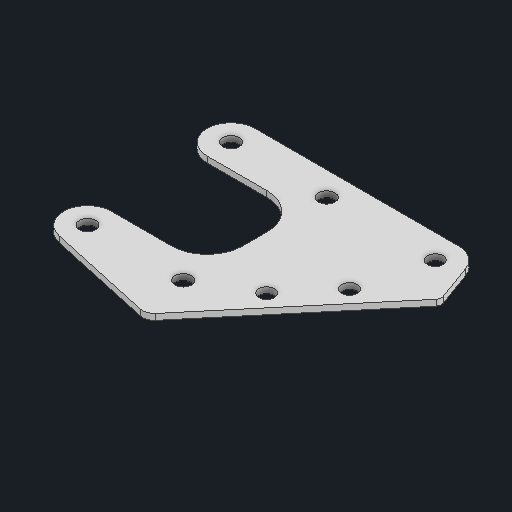
# Autodesk Inventor part: funel_gusset
Saved by Autodesk Inventor 2025 (Build 290162000, 162)
## iProperties
Created: 2024-10-12
Part Number: funel_gusset
Material: Generic
Document SubType Name: Modeling
Designer: Averey Ku
Density: 1 g/cm^3
Appearance: Default
d0: 0.164 in
d1: 0.500 in
d6: 0.375 in
d8: 0.164 in
d9: 0.063 in
d14: 0.164 in
d15: 0.615 in
d17: 0.125 in
Author: Averey Ku
Autodesk Inventor part; units mm, degrees
ref_plane "YZ Plane" through (0, 0, 0) normal (1, 0, 0) x (0, 1, 0)
ref_plane "XZ Plane" through (0, 0, 0) normal (0, 1, 0) x (-1, 0, 0)
ref_plane "XY Plane" through (0, 0, 0) normal (0, 0, 1) x (1, 0, 0)
sketch "main" plane through (0, 0, 0) normal (0, 0, 1) x (1, 0, 0)
  circle A0 centre (-18.9483, -3.9137) radius 2.0828
  arc A1 (-24.9153, -6.0856) -> (-18.95, -10.2637) centre (-18.9483, -3.9137) ccw
  line L0 (5.8565, 45.4052) -> (-28.0879, 4.9518)
  circle A2 centre (9.8531, -3.9215) radius 2.1844
  line L1 (-18.95, -10.2637) -> (35.2514, -10.2783)
  line L2 (9.8472, 18.301) -> (9.8489, 11.9535)
  arc A3 (9.8489, 11.9535) -> (19.3764, 2.4311) centre (19.3739, 11.9561) ccw
  circle A4 centre (9.8531, 34.1785) radius 2.1844
  line L3 (35.2514, 2.4354) -> (19.3764, 2.4311)
  arc A5 (35.2514, -10.2783) -> (35.2514, 2.4354) centre (35.2531, -3.9215) ccw
  circle A6 centre (35.2531, 34.1785) radius 2.1844
  arc A7 (35.2531, 27.8285) -> (36.6181, 40.3801) centre (35.2531, 34.1785) ccw
  circle A8 centre (35.2531, -3.9215) radius 2.1844
  line L4 (-28.3636, 3.3884) -> (-24.9153, -6.0856)
  line L5 (19.3722, 27.8285) -> (35.2531, 27.8285)
  arc A9 (19.3722, 27.8285) -> (9.8472, 18.301) centre (19.3722, 18.3035) ccw
  circle A10 centre (-14.2094, 14.0824) radius 2.0828
  arc A11 (-28.0879, 4.9518) -> (-28.3636, 3.3884) centre (-26.8718, 3.9314) ccw
  circle A12 centre (-4.1684, 26.0488) radius 2.0828
  line L6 (-4.1684, 26.0488) -> (-14.2094, 14.0824)
  line L7 (8.9712, 46.4651) -> (36.6181, 40.3801)
  arc A13 (8.9712, 46.4651) -> (5.8565, 45.4052) centre (8.2887, 43.3643) ccw
  point P0 (9.379, 13.4106)
  point P1 (9.8514, 2.4285)
  point P2 (9.8446, 27.8285)
  dimension "d0" = 4.1656
  dimension "d1" = 12.7
  dimension "d6" = 9.525
  dimension "d8" = 4.1656
  dimension "d9" = 1.5875
  dimension "d14" = 4.1656
  dimension "d15" = 15.621
  dimension "d17" = 3.175
  measures "d0" diameter of A0
  measures "d1" diameter of A1
  measures "d6" radius of A9
  measures "d8" diameter of A10
  measures "d9" radius of A11
  measures "d14" diameter of A12
  measures "d15" distance of L6.start L6.end
  measures "d17" radius of A13
sketch "Sketch1" plane through (0, 0, 0) normal (0, 1, 0) x (-1, 0, 0)
  circle A0 centre (-54.2014, -38.0923) radius 2.0828
  arc A1 (-60.1685, -40.2641) -> (-54.2031, -44.4423) centre (-54.2014, -38.0923) ccw
  line L0 (-29.3966, 11.2266) -> (-63.341, -29.2268)
  circle A2 centre (-25.4, -38.1) radius 2.1844
  line L1 (-54.2031, -44.4423) -> (-0.0017, -44.4568)
  line L2 (-25.406, -15.8776) -> (-25.4043, -22.225)
  arc A3 (-25.4043, -22.225) -> (-15.8767, -31.7474) centre (-15.8793, -22.2224) ccw
  circle A4 centre (-25.4, 0) radius 2.1844
  line L3 (-0.0017, -31.7432) -> (-15.8767, -31.7474)
  arc A5 (-0.0017, -44.4568) -> (-0.0017, -31.7432) centre (0, -38.1) ccw
  circle A6 centre (0, 0) radius 2.1844
  arc A7 (0, -6.35) -> (1.3649, 6.2016) centre (0, 0) ccw
  circle A8 centre (0, -38.1) radius 2.1844
  line L4 (-63.6167, -30.7901) -> (-60.1685, -40.2641)
  line L5 (-15.881, -6.35) -> (0, -6.35)
  arc A9 (-15.881, -6.35) -> (-25.406, -15.8776) centre (-15.881, -15.875) ccw
  circle A10 centre (-49.4625, -20.0961) radius 2.0828
  arc A11 (-63.341, -29.2268) -> (-63.6167, -30.7901) centre (-62.1249, -30.2472) ccw
  circle A12 centre (-39.4215, -8.1298) radius 2.0828
  line L6 (-39.4215, -8.1298) -> (-49.4625, -20.0961)
  line L7 (-26.2819, 12.2866) -> (1.3649, 6.2016)
  arc A13 (-26.2819, 12.2866) -> (-29.3966, 11.2266) centre (-26.9644, 9.1858) ccw
  constraints: 1 other
extrude "Extrusion1" add sketch "Sketch1" along normal blind 1.5875
body "Solid1"
